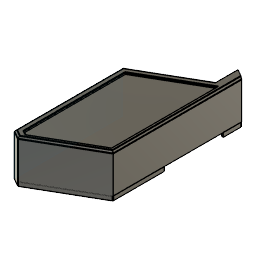
power-module-cover (Autodesk Fusion 360 design; units mm, degrees)
part number: 2026-08-04-16-25-20-525
Autodesk Fusion 360 part; units mm, degrees
sketch "Sketch1" plane through (0, 0, 0) normal (0, 0, 1) x (1, 0, 0)
  arc A0 (86.2786, -26.0102) -> (86.7786, -25.1442) centre (85.7786, -25.1442) ccw
  line L0 (86.7786, 34.1693) -> (82.7786, 34.1693)
  arc A1 (6.4015, -60.3646) -> (6.9015, -61.2307) centre (7.4015, -60.3646) ccw
  arc A2 (6.9015, 65.8993) -> (6.4015, 65.0333) centre (7.4015, 65.0333) ccw
  arc A3 (15.5882, -66.246) -> (16.5882, -66.246) centre (16.0882, -65.3799) ccw
  line L1 (6.9015, -61.2307) -> (15.5882, -66.246)
  line L2 (10.4015, -58.6326) -> (10.4015, 63.3013)
  line L3 (8.5355, -59.7099) -> (8.5355, 64.5333)
  line L4 (16.0882, -61.9158) -> (10.4015, -58.6326)
  line L5 (16.5882, -66.246) -> (86.2786, -26.0102)
  line L6 (86.9126, -25.6442) -> (16.2222, -66.4573)
  line L7 (78.8872, 105.1509) -> (78.8872, 126.6799)
  line L8 (82.7786, 34.1693) -> (82.7786, -23.4121)
  line L9 (6.5355, -60.8646) -> (16.2222, -66.4573)
  line L10 (78.8872, 126.6799) -> (84.9126, 123.2011)
  line L11 (86.9126, 124.3558) -> (86.9126, -25.6442)
  line L12 (84.9126, -24.4895) -> (16.2222, -64.1479)
  line L13 (8.5355, -59.7099) -> (16.2222, -64.1479)
  line L14 (6.4015, 65.0333) -> (6.4015, -60.3646)
  line L15 (86.7786, -25.1442) -> (86.7786, 34.1693)
  line L16 (82.7786, -23.4121) -> (16.0882, -61.9158)
  line L17 (8.5355, 64.5333) -> (78.8872, 105.1509)
  arc A4 (86.7786, 123.7011) -> (86.2786, 124.5671) centre (85.7786, 123.7011) ccw
  arc A5 (76.2532, 105.9396) -> (76.7532, 106.8056) centre (75.7532, 106.8056) ccw
  line L18 (76.2532, 105.9396) -> (6.9015, 65.8993)
  line L19 (6.5355, -60.8646) -> (6.5355, 65.688)
  line L20 (6.5355, 65.688) -> (76.8872, 106.3056)
  line L21 (76.8872, 106.3056) -> (76.8872, 130.144)
  line L22 (84.9126, 123.2011) -> (84.9126, -24.4895)
  arc A6 (78.2532, 129.2006) -> (76.7532, 128.3346) centre (77.7532, 128.3346) ccw
  line L23 (76.7532, 128.3346) -> (76.7532, 106.8056)
  line L24 (86.2786, 124.5671) -> (78.2532, 129.2006)
  line L25 (76.8872, 130.144) -> (86.9126, 124.3558)
  line L26 (82.7786, 121.9691) -> (82.7786, 102.9365)
  line L27 (80.7532, 103.9188) -> (80.7532, 123.1384)
  line L28 (82.7786, 102.9365) -> (86.7786, 102.9365)
  line L29 (10.4015, 63.3013) -> (80.7532, 103.9188)
  line L30 (86.7786, 102.9365) -> (86.7786, 123.7011)
  line L31 (80.7532, 123.1384) -> (82.7786, 121.9691)
  point P0 (14.803, 130.0666)
  dimension "d1" = 2
  dimension "d2" = 150
  dimension "d3" = 126.5527
  dimension "d4" = 90.1865
  dimension "d5" = 80.3771
  dimension "d6" = 10.4015
  dimension "d7" = 58.6326
  dimension "d8" = 3.866
  dimension "d9" = 1
  dimension "d10" = 120
  dimension "d11" = 196.5942
  dimension "d12" = 121.9339
  dimension "d13" = 6.5665
  dimension "d14" = 4.4015
  dimension "d15" = 188.6992
  dimension "d16" = 92.8019
  dimension "d17" = 161.5691
  dimension "d18" = 4
  dimension "d19" = 5.6867
  dimension "d20" = 65.3517
  dimension "d21" = 67.3517
  dimension "d22" = 70.3517
  dimension "d23" = 72.3771
  dimension "d24" = 75.3771
  dimension "d25" = 5.8207
  dimension "d26" = 66.4857
  dimension "d27" = 196.6013
  dimension "d28" = 120
  dimension "d29" = 119.2846
  dimension "d30" = 4
  dimension "d31" = 76.3771
  dimension "d32" = 4
  constraint parallel L6 L20
  constraint parallel L11 L19
  constraint parallel L9 L25
  constraint tangent A5 L20
  constraint tangent A2 L20
  constraint tangent A3 L6
  constraint parallel L11 L21
  constraint equal L20 L29
  constraint tangent A2 L14
  constraint tangent A2 L18
  constraint tangent A3 L1
  constraint tangent A3 L5
  constraint tangent A5 L18
  constraint tangent A5 L23
  constraint tangent A6 L23
  constraint tangent A6 L24
  constraint tangent A4 L24
  constraint tangent A4 L30
  constraint parallel L4 L31
  constraint parallel L1 L4
  constraint parallel L2 L30
  constraint parallel L4 L24
  constraint equal A0 A2
  constraint equal A0 A3
  constraint equal A0 A5
  constraint equal A0 A6
  constraint equal A0 A4
  constraint midpoint L9.start A1
  constraint tangent A0 L6
  constraint coincident A0.start L6
  constraint tangent A1 L14
  constraint parallel L16 L18
  constraint parallel L15 L23
  constraint perpendicular L28 L30
  constraint collinear L15 L30
  constraint tangent A0 L15
  measures "d2" distance of L6.start L11.start
  measures "d3" distance of L9.start L19.end
  measures "d4" distance of L11.start L0
  measures "d5" distance of L11 L19
  measures "d6" distance of origin L2
  measures "d7" vertical distance of origin L2.start
  measures "d8" distance of L2 L19
  measures "d9" radius of A3
  measures "d10" angle of L2 L4
  measures "d11" distance of L4 L24
  measures "d12" vertical distance of L2.start L2.end
  measures "d13" distance of L4.start L2.start
  measures "d14" distance of P0 L2
  measures "d15" vertical distance of P0 L2.start
  measures "d16" distance of L2.start L0
  measures "d17" distance of L2.start L28
  measures "d18" distance of L2 L14
  measures "d19" distance of A3.centre L2
  measures "d20" distance of A5.centre L2
  measures "d21" distance of A6.centre L2
  measures "d22" distance of L2 L27
  measures "d23" distance of L2 L26
  measures "d24" distance of A4.centre L2
  measures "d25" distance of L6.end L2
  measures "d26" distance of L2 L21
  measures "d27" vertical distance of L21.end L6.end
  measures "d28" angle of L9 L19
  measures "d29" distance of L6 L20
  measures "d30" distance of L20 L29
  measures "d31" distance of L8 L14
  measures "d32" distance of L24 L31
extrude "Extrude1" add sketch "Sketch1" against normal blind 5 contours A0 L0 A2 A3 L3 L5 L6 L7 L9 L10 L12 L13 L15 L17 A4 L18 L19 L20 L21 L22 A6 L24 L28 L30
sketch "Sketch2" plane through (31.8324, -55.1353, 0) normal (-0.5, 0.866025, 0) x (-0.866025, -0.5, 0)
  line L0 (18.0251, 0) -> (-61.2917, 0)
  line L1 (-61.2917, 0) -> (-61.2917, -5)
  line L2 (-61.2917, -5) -> (18.0251, -5)
  line L3 (18.0251, -5) -> (18.0251, 0)
  line L4 (-61.2917, -0.8) -> (18.0251, -0.8)
  dimension "d35" = 0.8
  constraint coincident L1 L4.start
  constraint coincident L3 L4.end
  constraint perpendicular L3 L4
  measures "d35" distance of L0 L4
extrude "Extrude2" cut sketch "Sketch2" against normal blind 1.3 contours L0 L1 L3 L4
sketch "Sketch3" plane through (-25.8099, 44.704, 0) normal (0.5, -0.866025, 0) x (0.866025, 0.5, 0)
  line L0 (120.8938, 0) -> (39.6586, 0)
  line L1 (39.6586, 0) -> (39.6586, -5)
  line L2 (39.6586, -5) -> (120.8938, -5)
  line L3 (120.8938, -5) -> (120.8938, 0)
  line L4 (39.6586, -1) -> (120.8938, -1)
  dimension "d38" = 1
  constraint coincident L1 L4.start
  constraint coincident L3 L4.end
  constraint perpendicular L3 L4
  measures "d38" distance of L0 L4
extrude "Extrude3" cut sketch "Sketch3" against normal blind 1.5 contours L0 L1 L3 L4
sketch "Sketch4" plane through (0, 0, 0) normal (0, 0, 1) x (1, 0, 0)
  arc A0 (86.2786, -26.0102) -> (86.7786, -25.1442) centre (85.7786, -25.1442) ccw
  line L0 (86.7786, 34.1693) -> (82.7786, 34.1693)
  arc A1 (6.4015, -60.3646) -> (6.9015, -61.2307) centre (7.4015, -60.3646) ccw
  arc A2 (6.9015, 65.8993) -> (6.4015, 65.0333) centre (7.4015, 65.0333) ccw
  arc A3 (15.5882, -66.246) -> (16.5882, -66.246) centre (16.0882, -65.3799) ccw
  line L1 (6.9015, -61.2307) -> (15.5882, -66.246)
  line L2 (10.4015, -58.6326) -> (10.4015, 63.3013)
  line L3 (8.5355, -59.7099) -> (8.5355, 64.5333)
  line L4 (16.0882, -61.9158) -> (10.4015, -58.6326)
  line L5 (16.5882, -66.246) -> (86.2786, -26.0102)
  line L6 (86.9126, -25.6442) -> (16.2222, -66.4573)
  line L7 (78.8872, 105.1509) -> (78.8872, 126.6799)
  line L8 (82.7786, 34.1693) -> (82.7786, -23.4121)
  line L9 (6.5355, -60.8646) -> (16.2222, -66.4573)
  line L10 (78.8872, 126.6799) -> (84.9126, 123.2011)
  line L11 (86.9126, 124.3558) -> (86.9126, -25.6442)
  line L12 (84.9126, -24.4895) -> (16.2222, -64.1479)
  line L13 (8.5355, -59.7099) -> (16.2222, -64.1479)
  line L14 (6.4015, 65.0333) -> (6.4015, -60.3646)
  line L15 (86.7786, -25.1442) -> (86.7786, 34.1693)
  line L16 (82.7786, -23.4121) -> (16.0882, -61.9158)
  line L17 (8.5355, 64.5333) -> (78.8872, 105.1509)
  arc A4 (86.7786, 123.7011) -> (86.2786, 124.5671) centre (85.7786, 123.7011) ccw
  arc A5 (76.2532, 105.9396) -> (76.7532, 106.8056) centre (75.7532, 106.8056) ccw
  line L18 (76.2532, 105.9396) -> (6.9015, 65.8993)
  line L19 (6.5355, -60.8646) -> (6.5355, 65.688)
  line L20 (6.5355, 65.688) -> (76.8872, 106.3056)
  line L21 (76.8872, 106.3056) -> (76.8872, 130.144)
  line L22 (84.9126, 123.2011) -> (84.9126, -24.4895)
  arc A6 (78.2532, 129.2006) -> (76.7532, 128.3346) centre (77.7532, 128.3346) ccw
  line L23 (76.7532, 128.3346) -> (76.7532, 106.8056)
  line L24 (86.2786, 124.5671) -> (78.2532, 129.2006)
  line L25 (76.8872, 130.144) -> (86.9126, 124.3558)
  line L26 (82.7786, 121.9691) -> (82.7786, 102.9365)
  line L27 (80.7532, 103.9188) -> (80.7532, 123.1384)
  line L28 (82.7786, 102.9365) -> (86.7786, 102.9365)
  line L29 (10.4015, 63.3013) -> (80.7532, 103.9188)
  line L30 (86.7786, 102.9365) -> (86.7786, 123.7011)
  line L31 (80.7532, 123.1384) -> (82.7786, 121.9691)
  point P0 (14.803, 130.0666)
  dimension "d41" = 2
  dimension "d42" = 150
  dimension "d43" = 126.5527
  dimension "d44" = 90.1865
  dimension "d45" = 80.3771
  dimension "d46" = 10.4015
  dimension "d47" = 3.866
  dimension "d48" = 1
  dimension "d49" = 80.3771
  dimension "d50" = 120
  dimension "d51" = 120
  dimension "d52" = 4
  dimension "d53" = 115.2846
  dimension "d54" = 119.2846
  dimension "d55" = 4
  dimension "d56" = 196.5942
  dimension "d57" = 200.5942
  dimension "d58" = 20.7646
  dimension "d59" = 4
  dimension "d60" = 4.4015
  dimension "d61" = 188.6992
  constraint parallel L6 L20
  constraint parallel L11 L19
  constraint parallel L9 L25
  constraint tangent A5 L20
  constraint tangent A2 L20
  constraint tangent A3 L6
  constraint parallel L11 L21
  constraint equal L20 L29
  constraint tangent A1 L14
  constraint tangent A2 L14
  constraint tangent A1 L1
  constraint tangent A2 L18
  constraint tangent A3 L1
  constraint tangent A3 L5
  constraint tangent A5 L18
  constraint tangent A5 L23
  constraint tangent A6 L23
  constraint tangent A6 L24
  constraint tangent A0 L5
  constraint tangent A4 L24
  constraint tangent A0 L15
  constraint tangent A4 L30
  constraint tangent A0 L6
  constraint coincident A0.start L6
  constraint coincident A2.start L20
  constraint perpendicular L28 L30
  constraint perpendicular L26 L28
  constraint perpendicular L0 L8
  constraint perpendicular L0 L15
  constraint parallel L23 L26
  constraint parallel L8 L23
  constraint parallel L4 L31
  constraint parallel L8 L27
  constraint parallel L16 L29
  constraint parallel L1 L4
  constraint parallel L5 L16
  constraint parallel L8 L14
  constraint parallel L4 L24
  constraint parallel L2 L8
  constraint collinear L8 L26
  constraint collinear L15 L30
  constraint vertical L14
  constraint vertical L19
  constraint vertical L6.end L12.end
  constraint equal A0 A1
  constraint equal A0 A2
  constraint equal A0 A3
  constraint equal A0 A4
  constraint equal A0 A5
  constraint equal A0 A6
  constraint equal L7 L23
  constraint midpoint L9.start A1
  measures "d42" distance of L6.start L11.start
  measures "d43" distance of L9.start L19.end
  measures "d44" distance of L11.start L0
  measures "d45" distance of L11 L19
  measures "d46" distance of origin L2
  measures "d47" distance of L2 L19
  measures "d48" radius of A3
  measures "d49" distance of L14 L30
  measures "d50" angle of L2 L4
  measures "d51" angle of L9 L19
  measures "d52" distance of L18 L29
  measures "d53" distance of L16 L18
  measures "d54" distance of L5 L18
  measures "d55" distance of L24 L31
  measures "d56" distance of L4 L24
  measures "d57" distance of L1 L24
  measures "d58" distance of A4.centre L28
  measures "d59" distance of L26 L30
  measures "d60" distance of P0 L2
  measures "d61" vertical distance of P0 L2.start
extrude "Extrude4" add sketch "Sketch4" along normal blind 45 contours A0 L0 A2 A3 L3 L5 L6 L7 L9 L10 L12 L13 L15 L17 A4 L18 L19 L20 L21 L22 A6 L24 L28 L30 | A0 L0 L6 L11 L15 A4 L21 L22 A6 L24 L25 L28 L30 | L0 L2 L3 L4 L7 L8 L10 L12 L13 L16 L17 L22 L26 L27 L28 L29 L31
sketch "Sketch5" plane through (0, 0, 45) normal (0, 0, 1) x (-1, 0, 0)
  line L0 (-80.7532, -103.9188) -> (-80.7532, -123.1384)
  line L1 (-80.7532, -123.1384) -> (-82.7786, -121.9691)
  line L2 (-82.7786, -121.9691) -> (-82.7786, -102.9365)
  line L3 (-82.7786, -102.9365) -> (-84.9126, -102.9365)
  line L4 (-84.9126, -102.9365) -> (-84.9126, -34.1693)
  line L5 (-84.9126, -34.1693) -> (-82.7786, -34.1693)
  line L6 (-82.7786, -34.1693) -> (-82.7786, 23.4121)
  line L7 (-82.7786, 23.4121) -> (-16.0882, 61.9158)
  line L8 (-16.0882, 61.9158) -> (-10.4015, 58.6326)
  line L9 (-10.4015, 58.6326) -> (-10.4015, -63.3013)
  line L10 (-10.4015, -63.3013) -> (-80.7532, -103.9188)
  line L11 (-86.9126, 25.6442) -> (-86.9126, -124.3558)
  line L12 (-86.9126, -124.3558) -> (-76.8872, -130.144)
  line L13 (-76.8872, -130.144) -> (-76.8872, -106.3056)
  line L14 (-76.8872, -106.3056) -> (-6.9015, -65.8993)
  line L15 (-6.5355, -65.5333) -> (-6.5355, 60.8646)
  line L16 (-6.5355, 60.8646) -> (-16.0882, 66.3799)
  arc A0 (-16.0882, 66.3799) -> (-16.5882, 66.246) centre (-16.0882, 65.3799) ccw
  line L17 (-16.5882, 66.246) -> (-86.9126, 25.6442)
  line L18 (-82.7786, 23.4121) -> (-16.0882, 61.9158)
  line L19 (-10.4015, 58.6326) -> (-10.4015, -63.3013)
  line L20 (-80.7532, -103.9188) -> (-80.7532, -123.1384)
  line L21 (-82.7786, -121.9691) -> (-82.7786, -102.9365)
  line L22 (-84.9126, -102.9365) -> (-84.9126, -34.1693)
  line L23 (-82.7786, -34.1693) -> (-82.7786, 23.4121)
  arc A1 (-6.9015, -65.8993) -> (-6.5355, -65.5333) centre (-7.4015, -65.0333) ccw
  constraint coincident L6.end L7.start
  constraint coincident L7.end L8.start
  constraint coincident L8.end L9.start
  constraint coincident L9.end L10.start
  constraint coincident L0.start L10.end
  constraint coincident L0.end L1.start
  constraint coincident L1.end L2.start
  constraint coincident L2.end L3.start
  constraint coincident L3.end L4.start
  constraint coincident L4.end L5.start
  constraint coincident L5.end L6.start
extrude "Extrude5" add sketch "Sketch5" against normal blind 5 contours L0 L1 L2 L3 L4 L5 L6 L7 L8 L9 L10 L18 L19 L20 L21 L22 L23
chamfer "Chamfer1" distance 2 angle 45 1 edges at (6.5355, 2.3343, 45) tangent chain off
chamfer "Chamfer2" distance 2 angle 45 1 edges at (42.7113, 86.5742, 45) tangent chain off
chamfer "Chamfer3" distance 2 angle 45 1 edges at (12.3119, -64.1996, 45) tangent chain off
sketch "Sketch9" plane through (0, 0, 45) normal (0, 0, 1) x (-1, 0, 0)
  line L0 (-8.5355, 59.7099) -> (-18.2222, 65.3026)
  line L1 (-18.2222, 65.3026) -> (-86.9126, 25.6442)
  line L2 (-86.9126, 25.6442) -> (-86.9126, -124.3558)
  line L3 (-86.9126, -124.3558) -> (-76.8872, -130.144)
  line L4 (-76.8872, -130.144) -> (-76.8872, -103.9962)
  line L5 (-76.8872, -103.9962) -> (-8.5355, -64.5333)
  line L6 (-8.5355, -64.5333) -> (-8.5355, 59.7099)
  line L7 (-81.8872, -101.1094) -> (-13.5355, -61.6466)
  line L8 (-13.5355, -61.6466) -> (-13.5355, 56.8232)
  line L9 (-13.5355, 56.8232) -> (-18.2222, 59.5291)
  line L10 (-18.2222, 59.5291) -> (-81.9126, 22.7574)
  line L11 (-81.9126, -121.4691) -> (-81.8872, -121.4837)
  line L12 (-81.8872, -101.1094) -> (-81.9126, 22.7574)
  dimension "d157" = -5
  dimension "d158" = 5.0254
  dimension "d159" = 5
  dimension "d160" = 0.012
  measures "d158" distance of L2 L11.end
  measures "d159" distance of L2 L10.end
  measures "d160" angle of L4 L12
extrude "Extrude10" cut sketch "Sketch9" against normal blind 1.5 contours L7 L8 L9 L10 L12
chamfer "Chamfer4" distance 0.8 angle 45 5 edges at (81.8999, 39.176, 43.5) (50.0674, -41.1433, 43.5) (47.7113, 81.378, 43.5) (13.5355, 2.4117, 43.5) (15.8788, -58.1761, 43.5) tangent chain off
chamfer "Chamfer5" distance 0.5 angle 45 5 edges at (81.8999, 39.176, 45) (50.0674, -41.1433, 45) (15.8788, -58.1761, 45) (13.5355, 2.4117, 45) (47.7113, 81.378, 45) tangent chain off
chamfer "Chamfer6" distance 2 angle 45 1 edges at (52.5674, -45.4734, 45) tangent chain off
chamfer "Chamfer7" distance 2 angle 45 1 edges at (86.9126, 50.5105, 45) tangent chain off
sketch "Sketch10" plane through (-26.8099, 46.4361, 0) normal (-0.5, 0.866025, 0) x (-0.866025, -0.5, 0)
  line L0 (-38.9265, 43) -> (-119.7391, 43)
  line L1 (-119.7391, 43) -> (-119.7391, -5)
  line L2 (-119.7391, -5) -> (-38.9265, -5)
  line L3 (-38.9265, -5) -> (-38.9265, 43)
  line L4 (-100, 25) -> (-74.9959, 25)
  line L5 (-74.9959, 25) -> (-74.9959, 18.1077)
  line L6 (-74.9959, 18.1077) -> (-100, 18.1077)
  line L7 (-100, 18.1077) -> (-100, 25)
  dimension "d167" = 44.7431
  dimension "d168" = 23.1077
  dimension "d169" = 6.8923
  dimension "d170" = 25.0041
  constraint horizontal L4
  constraint vertical L5
  constraint horizontal L6
  constraint vertical L7
  measures "d167" distance of L1 L5
  measures "d168" distance of L2 L6
  measures "d169" distance of L4 L6
  measures "d170" distance of L5 L7
extrude "Extrude11" cut sketch "Sketch10" against normal blind 15 contours L4 L5 L6 L7
fillet "Fillet4" radius 0.8 5 edges at (8.5355, 2.4117, 45) (42.7113, 84.2648, 45) (84.9126, 50.5105, 45) (50.5674, -44.3187, 45) (12.3788, -61.9289, 45)
fillet "Fillet5" radius 0.8 7 edges at (41.8943, 86.1025, 43) (6.7435, 65.7863, 43.0189) (6.5355, 2.3343, 43) (11.3119, -63.6223, 43) (16.4113, -66.3263, 43.0189) (51.7504, -45.9451, 43) (86.9126, 49.3558, 43)
sketch "Sketch11" plane through (6.5355, 0, 0) normal (-1, 0, 0) x (0, -1, 0)
  line L0 (60.8646, 42.6686) -> (-65.5333, 42.6686)
  line L1 (-65.5333, 42.6686) -> (-65.5333, -5)
  line L2 (-65.5333, -5) -> (60.8646, -5)
  line L3 (60.8646, -5) -> (60.8646, 42.6686)
sketch "Sketch12" plane through (6.5355, 0, 0) normal (-1, 0, 0) x (0, -1, 0)
  line L0 (-61.5333, 40.1686) -> (56.8646, 40.1686)
  line L1 (58.3646, 38.6686) -> (58.3646, -1)
  line L2 (56.8646, -2.5) -> (-61.5333, -2.5)
  line L3 (-63.0333, -1) -> (-63.0333, 38.6686)
  line L4 (-65.5333, 42.6686) -> (-65.5333, -5)
  line L5 (60.8646, -5) -> (60.8646, 42.6686)
  line L6 (60.8646, 42.6686) -> (-65.5333, 42.6686)
  line L7 (-65.5333, -5) -> (60.8646, -5)
  line L8 (56.8646, 40.1686) -> (58.3646, 38.6686)
  line L9 (-61.5333, 40.1686) -> (-63.0333, 38.6686)
  line L10 (58.3646, -1) -> (56.8646, -2.5)
  line L11 (-63.0333, -1) -> (-61.5333, -2.5)
  point P0 (-63.0333, 40.1686)
  point P1 (58.3646, 40.1686)
  point P2 (58.3646, -2.5)
  point P3 (-63.0333, -2.5)
  dimension "d177" = 2.5
  dimension "d178" = 2.5
  dimension "d179" = 2.5
  dimension "d180" = 2.5
  dimension "d183" = 1.5
  dimension "d184" = 1.5
  dimension "d185" = 1.5
  dimension "d186" = 1.5
  dimension "d187" = 1.5
  dimension "d188" = 1.5
  dimension "d189" = 1.5
  dimension "d190" = 1.5
  constraint horizontal L0
  constraint vertical L1
  constraint horizontal L2
  constraint vertical L3
  constraint coincident P1 L0
  constraint coincident P1 L1
  constraint coincident P0 L0
  constraint coincident P0 L3
  constraint coincident P2 L1
  constraint coincident P2 L2
  constraint coincident P3 L3
  constraint coincident P3 L2
  measures "d177" distance of L3 L4
  measures "d178" distance of L1 L5
  measures "d179" distance of L0 L6
  measures "d180" distance of L2 L7
  measures "d183" distance of P1 L0.end
  measures "d184" distance of P1 L1.start
  measures "d185" distance of P0 L0.start
  measures "d186" distance of P0 L3.end
  measures "d187" distance of P2 L1.end
  measures "d188" distance of P2 L2.start
  measures "d189" distance of P3 L3.start
  measures "d190" distance of P3 L2.end
extrude "Extrude12" cut sketch "Sketch12" against normal blind 1.5 contours L0 L1 L2 L3 L8 L9 L10 L11
chamfer "Chamfer8" distance 1.2 angle 45 8 edges at (6.5355, 2.3343, -2.5) (6.5355, 2.3343, 40.1686) (6.5355, 63.0333, 18.8343) (6.5355, -58.3646, 18.8343) (6.5355, 62.2833, 39.4186) (6.5355, -57.6146, 39.4186) (6.5355, -57.6146, -1.75) (6.5355, 62.2833, -1.75) tangent chain off
equation "d184 = d183"
equation "d186 = d185"
equation "d188 = d187"
